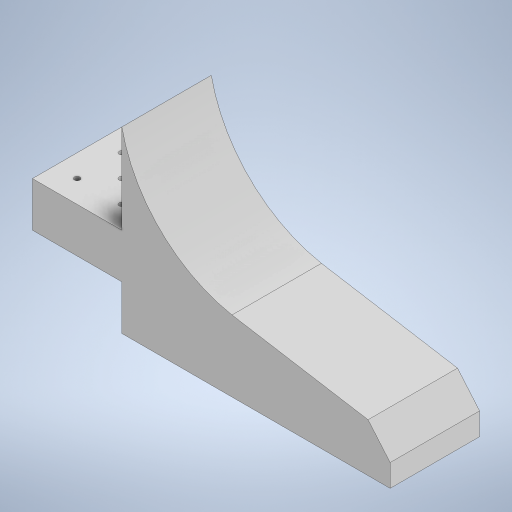
# Autodesk Inventor part: Table foot X4
Saved by Autodesk Inventor 2023 (Build 270158000, 158)
## iProperties
Created: 2022-11-23
Part Number: Table foot X4
Material: Generic
Document SubType Name: Modeling
Designer: surat
Density: 1 g/cm^3
Appearance: Default
Author: surat
Autodesk Inventor part; units mm, degrees
ref_plane "YZ Plane" through (0, 0, 0) normal (1, 0, 0) x (0, 1, 0)
ref_plane "XZ Plane" through (0, 0, 0) normal (0, 1, 0) x (-1, 0, 0)
ref_plane "XY Plane" through (0, 0, 0) normal (0, 0, 1) x (1, 0, 0)
sketch "Sketch1" plane through (0, 0, 0) normal (0, 0, 1) x (1, 0, 0)
  line L0 (0, 0) -> (406.4, 0)
  line L1 (406.4, 0) -> (406.4, 203.2)
  line L2 (406.4, 203.2) -> (0, 203.2)
  line L3 (0, 203.2) -> (0, 0)
  line L4 (0, 101.6) -> (664.7751, 101.6)
  line L5 (101.6, 101.6) -> (406.4, 50.8)
  line L6 (0, 50.8) -> (101.6, 50.8)
  line L7 (101.6, 50.8) -> (101.6, 0)
  line L8 (101.6, 101.6) -> (101.6, 203.2)
  arc A0 (101.6, 203.2) -> (233.5206, 79.6132) centre (256.07, 235.8848) ccw
  point P0 (226.7178, 80.747)
  dimension "d0" = 406.4
  dimension "d1" = 203.2
  dimension "d2" = 101.6
  dimension "d3" = 50.8
  dimension "d26" = 101.6
  constraints: 18 end point, 6 point on line, 3 horizontal, 2 parallel, 2 perpendicular, 2 point on circle, 1 centre point, 1 midpoint
  measures "d0" distance of L2.end L1.end
  measures "d1" distance of L1.end L0.end
  measures "d2" distance of L5.start L4.start
  measures "d3" distance of L0.end L5.end
  measures "d26" distance of L5.start L8.end
extrude "Extrusion1" add sketch "Sketch1" along normal blind 101.6 contours L7 L6 L3 L4 L5 A0 L1 L0 | L8 A0 L4 | L4 A0 L5 | A0 L5
chamfer "Chamfer1" distance 25.4 angle 45 1 edges at (406.4, 50.8, 50.8)
sketch "Sketch2" plane through (0, 50.8, 0) normal (0, -1, 0) x (1, 0, 0)
  circle A0 centre (25.4, 76.2) radius 3.175
  circle A1 centre (76.2, 76.2) radius 3.175
  circle A2 centre (76.2, 25.4) radius 3.175
  circle A3 centre (50.8, 50.8) radius 3.175
  circle A4 centre (25.4, 25.4) radius 3.175
  line L0 (0, 101.6) -> (101.6, 101.6) projected
  line L1 (0, 0) -> (0, 101.6) projected
  line L2 (101.6, 0) -> (101.6, 101.6) projected
  line L3 (0, 0) -> (101.6, 0) projected
  dimension "d9" = 6.35
  dimension "d10" = 6.35
  dimension "d11" = 6.35
  dimension "d12" = 6.35
  dimension "d13" = 6.35
  dimension "d14" = 25.4
  dimension "d15" = 25.4
  dimension "d16" = 25.4
  dimension "d17" = 25.4
  dimension "d18" = 25.4
  dimension "d19" = 25.4
  dimension "d20" = 25.4
  dimension "d21" = 25.4
  dimension "d22" = 50.8
  dimension "d23" = 50.8
  constraints: 5 centre point
  measures "d9" diameter of A0
  measures "d10" diameter of A1
  measures "d11" diameter of A2
  measures "d12" diameter of A3
  measures "d13" diameter of A4
  measures "d14" distance from line of L0 A0.centre
  measures "d15" distance from line of L1 A0.centre
  measures "d16" distance from line of L0 A1.centre
  measures "d17" distance from line of L2 A1.centre
  measures "d18" distance from line of L3 A2.centre
  measures "d19" distance from line of L2 A2.centre
  measures "d20" distance from line of L1 A4.centre
  measures "d21" distance from line of L3 A4.centre
  measures "d22" distance from line of L0 A3.centre
  measures "d23" distance from line of L2 A3.centre
extrude "Extrusion2" cut sketch "Sketch2" against normal blind 101.6 contours A0 | A1 | A2 | A3 | A4
body "Solid1"
